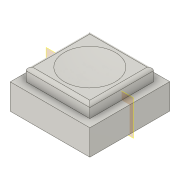
# Autodesk Inventor part: Top Button
Saved by Autodesk Inventor 2019 (Build 230136000, 136)
## iProperties
Created: 2019-03-17
Part Number: Top Button
Material: PC/ABS Plastic
Document SubType Name: Modeling
Designer: Jared
Density: 0.357273 g/cm^3
Appearance: Steel
Author: Jared
Autodesk Inventor part; units mm, degrees
ref_plane "YZ Plane" through (0, 0, 0) normal (1, 0, 0) x (0, 1, 0)
ref_plane "XZ Plane" through (0, 0, 0) normal (0, 1, 0) x (-1, 0, 0)
ref_plane "XY Plane" through (0, 0, 0) normal (0, 0, 1) x (1, 0, 0)
sketch "Sketch1" plane through (0, 0, 0) normal (0, 1, 0) x (-1, 0, 0)
  line L0 (0, 0) -> (12.5, 0)
  line L1 (12.5, 0) -> (12.5, -12.55)
  line L2 (12.5, -12.55) -> (0, -12.55)
  line L3 (0, -12.55) -> (0, 0)
  dimension "d0" = 12.5
  dimension "d1" = 12.55
  constraints: 8 end point, 2 parallel, 1 horizontal, 1 perpendicular
  measures "d0" distance of L1.end L2.end
  measures "d1" distance of L0.end L1.end
extrude "Extrusion1" add sketch "Sketch1" along normal blind 4
sketch "Sketch2" plane through (0, 4, 0) normal (0, 1, 0) x (1, 0, 0)
  line L0 (-11.25, 1.25) -> (-1.25, 1.25)
  line L1 (-1.25, 1.25) -> (-1.25, 11.25)
  line L2 (-1.25, 11.25) -> (-11.25, 11.25)
  line L3 (-11.25, 11.25) -> (-11.25, 1.25)
  line L4 (-12.5, 0) -> (0, 0) projected
  line L5 (-12.5, 12.55) -> (-12.5, 0) projected
  dimension "d4" = 10
  dimension "d5" = 10
  dimension "d6" = 1.25
  dimension "d7" = 1.25
  constraints: 8 end point, 2 parallel, 1 horizontal, 1 perpendicular
  measures "d4" distance of L2.end L1.end
  measures "d5" distance of L1.end L0.end
  measures "d6" distance between parallel lines of L4 L0
  measures "d7" distance between parallel lines of L5 L3
extrude "Extrusion2" add sketch "Sketch2" along normal blind 2
ref_plane "Work Plane1" through (-11.25, 4, -6.25) normal (0, 0, 1) x (1, 0, 0)
sketch "Sketch3" plane through (-11.25, 4, -6.25) normal (0, 0, 1) x (1, 0, 0)
  line L0 (10, 0) -> (0, 0) projected
  line L1 (10, 0) -> (10, 2) projected
  line L2 (0, 2) -> (10, 2) projected
  line L3 (0, 0) -> (0, 2) projected
  line L4 (5, 2) -> (5, 1.5)
  line L5 (5, 2) -> (9, 2)
  line L6 (5, 2) -> (1, 2)
  arc A0 (1, 2) -> (9, 2) centre (5, 17.75) ccw
  point P0 (11.25, -4)
  dimension "d10" = 0.5
  dimension "d11" = 4
  dimension "d12" = 4
  constraints: 6 end point, 3 point on circle, 2 point on line, 1 centre point, 1 midpoint, 1 perpendicular
  measures "d10" distance of L4.start L4.end
  measures "d11" distance of L4.start L5.end
  measures "d12" distance of L4.start L6.end
revolve "Revolution1" cut sketch "Sketch3" angle 360 about axis through (-6.25, 6, -6.25) along (0, -1, 0) picked at (7.2273, 1.9076) contours A0 L4 L2
fillet "Fillet1" radius 0.5 4 edges at (-11.25, 6, -6.25) (-6.25, 6, -11.25) (-1.25, 6, -6.25) (-6.25, 6, -1.25)
body "Solid1"
